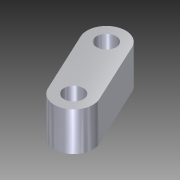
# Autodesk Inventor part: avstandsstykke
Saved by Autodesk Inventor 2015 (Build 190159000, 159)
## iProperties
Created: 2015-02-25
Part Number: avstandsstykke
Material: Generic
Document SubType Name: Modeling
Designer: janov_000
Density: 1 g/cm^3
Appearance: Aluminum - Flat
Author: janov_000
Autodesk Inventor part; units mm, degrees
ref_plane "YZ Plane" through (0, 0, 0) normal (1, 0, 0) x (0, 1, 0)
ref_plane "XZ Plane" through (0, 0, 0) normal (0, 1, 0) x (-1, 0, 0)
ref_plane "XY Plane" through (0, 0, 0) normal (0, 0, 1) x (1, 0, 0)
sketch "Sketch3" plane through (0, 0, 0) normal (0, 0, 1) x (1, 0, 0)
  line L0 (71.8451, -79.0914) -> (79.2409, -94.9518) construction
  line L1 (67.3136, -81.2045) -> (74.7094, -97.0649)
  line L2 (83.7725, -92.8387) -> (76.3766, -76.9783)
  arc A0 (76.3766, -76.9783) -> (67.3136, -81.2045) centre (71.8451, -79.0914) ccw
  arc A1 (74.7094, -97.0649) -> (83.7725, -92.8387) centre (79.2409, -94.9518) ccw
  line L3 (79.2409, -94.9518) -> (71.8451, -79.0914)
  point P0 (0, 0)
  point P1 (75.543, -87.0216)
  dimension "d16" = 10
  constraints: 10 end point, 4 point on circle, 4 tangent, 2 centre point, 2 equal length, 1 midpoint
  measures "d16" diameter of A1
extrude "Extrusion2" add sketch "Sketch3" along normal blind 10
sketch "Sketch4" plane through (0, 0, 10) normal (0, 0, 1) x (1, 0, 0)
  line L0 (67.3136, -81.2045) -> (74.7094, -97.0649) projected
  arc A0 (74.7094, -97.0649) -> (83.7725, -92.8387) centre (79.2409, -94.9518) ccw projected
  line L1 (83.7725, -92.8387) -> (76.3766, -76.9783) projected
  arc A1 (76.3766, -76.9783) -> (67.3136, -81.2045) centre (71.8451, -79.0914) ccw projected
  point P0 (0, 0)
  constraints: 2 coincident
hole "Hole1" at (71.8451, -79.0914, 10) at (79.2409, -94.9518, 10) direction (0, 0, -1) diameter 5 end through all
body "Solid2"
